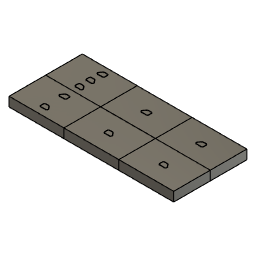
AD_mold_20200226_wide v4 (Autodesk Fusion 360 design; units mm, degrees)
Autodesk Fusion 360 part; units mm, degrees
note: some values were not read from the file. Chosen so that the rebuilt part matches the saved one: which bodies a step acts on.
sketch "Sketch1" plane through (0, 0, 0) normal (0, 1, 0) x (1, 0, 0)
  line L0 (-37.5181, 150.0315) -> (37.4819, 150.0315)
  line L1 (37.4819, 150.0315) -> (37.4819, -149.9685)
  line L2 (37.4819, -149.9685) -> (-37.5181, -149.9685)
  line L3 (-37.5181, -149.9685) -> (-37.5181, 150.0315)
  line L4 (-37.5181, -50.0913) -> (37.4819, -50.0913)
  line L5 (37.4819, -50.0913) -> (37.4819, -100.0913)
  line L6 (37.4819, -100.0913) -> (-37.5181, -100.0913)
  line L7 (-37.5181, -100.0913) -> (-37.5181, -50.0913)
  line L8 (-37.5181, -0.0913) -> (37.4819, -0.0913)
  line L9 (-37.5181, -50.0913) -> (-37.5181, -0.0913)
  line L10 (37.4819, -50.0913) -> (-37.5181, -50.0913)
  line L11 (37.4819, -0.0913) -> (37.4819, -50.0913)
  line L12 (37.4819, -100.0913) -> (-37.5181, -100.0913)
  line L13 (-37.5181, -150.0913) -> (-37.5181, -100.0913)
  line L14 (37.4819, -150.0913) -> (-37.5181, -150.0913)
  line L15 (37.4819, -100.0913) -> (37.4819, -150.0913)
  line L16 (-37.5181, 49.9087) -> (37.4819, 49.9087)
  line L17 (-37.5181, -0.0913) -> (-37.5181, 49.9087)
  line L18 (37.4819, -0.0913) -> (-37.5181, -0.0913)
  line L19 (37.4819, 49.9087) -> (37.4819, -0.0913)
  line L20 (-37.5181, 99.9087) -> (37.4819, 99.9087)
  line L21 (37.4819, 99.9087) -> (37.4819, 49.9087)
  line L22 (-37.5181, 49.9087) -> (37.4819, 49.9087)
  line L23 (-37.5181, 49.9087) -> (-37.5181, 99.9087)
  line L24 (37.4819, 149.9087) -> (37.4819, 99.9087)
  line L25 (-37.5181, 99.9087) -> (-37.5181, 149.9087)
  line L26 (-3.211, -128.2452) -> (3.289, -128.2452)
  arc A0 (3.289, -128.2452) -> (4.789, -126.7452) centre (3.289, -126.7452) ccw
  line L27 (4.789, -126.7452) -> (4.789, -123.3452)
  arc A1 (4.789, -123.3452) -> (3.289, -121.8452) centre (3.289, -123.3452) ccw
  line L28 (3.289, -121.8452) -> (-0.4902, -121.8452)
  arc A2 (-0.4902, -121.8452) -> (-1.6614, -122.408) centre (-0.4902, -123.3452) ccw
  line L29 (-4.3822, -125.808) -> (-1.6614, -122.408)
  arc A3 (-4.3822, -125.808) -> (-4.711, -126.7452) centre (-3.211, -126.7452) ccw
  arc A4 (-4.711, -126.7452) -> (-3.211, -128.2452) centre (-3.211, -126.7452) ccw
  line L30 (-3.211, -28.2452) -> (3.289, -28.2452)
  arc A5 (3.289, -28.2452) -> (4.789, -26.7452) centre (3.289, -26.7452) ccw
  line L31 (4.789, -26.7452) -> (4.789, -23.3452)
  arc A6 (4.789, -23.3452) -> (3.289, -21.8452) centre (3.289, -23.3452) ccw
  line L32 (3.289, -21.8452) -> (-0.4902, -21.8452)
  arc A7 (-0.4902, -21.8452) -> (-1.6614, -22.408) centre (-0.4902, -23.3452) ccw
  line L33 (-4.3822, -25.808) -> (-1.6614, -22.408)
  arc A8 (-4.3822, -25.808) -> (-4.711, -26.7452) centre (-3.211, -26.7452) ccw
  arc A9 (-4.711, -26.7452) -> (-3.211, -28.2452) centre (-3.211, -26.7452) ccw
  line L34 (4.789, 138.2548) -> (4.789, 141.6548)
  arc A10 (3.289, 136.7548) -> (4.789, 138.2548) centre (3.289, 138.2548) ccw
  line L35 (-3.211, 136.7548) -> (3.289, 136.7548)
  arc A11 (-4.711, 138.2548) -> (-3.211, 136.7548) centre (-3.211, 138.2548) ccw
  arc A12 (-4.3822, 139.192) -> (-4.711, 138.2548) centre (-3.211, 138.2548) ccw
  line L36 (-4.3822, 139.192) -> (-1.6614, 142.592)
  arc A13 (-0.4902, 143.1548) -> (-1.6614, 142.592) centre (-0.4902, 141.6548) ccw
  line L37 (3.289, 143.1548) -> (-0.4902, 143.1548)
  arc A14 (4.789, 141.6548) -> (3.289, 143.1548) centre (3.289, 141.6548) ccw
  line L38 (4.789, 86.2548) -> (4.789, 89.6548)
  arc A15 (3.289, 84.7548) -> (4.789, 86.2548) centre (3.289, 86.2548) ccw
  line L39 (-3.211, 84.7548) -> (3.289, 84.7548)
  arc A16 (-4.711, 86.2548) -> (-3.211, 84.7548) centre (-3.211, 86.2548) ccw
  arc A17 (-4.3822, 87.192) -> (-4.711, 86.2548) centre (-3.211, 86.2548) ccw
  line L40 (-4.3822, 87.192) -> (-1.6614, 90.592)
  arc A18 (-0.4902, 91.1548) -> (-1.6614, 90.592) centre (-0.4902, 89.6548) ccw
  line L41 (3.289, 91.1548) -> (-0.4902, 91.1548)
  arc A19 (4.789, 89.6548) -> (3.289, 91.1548) centre (3.289, 89.6548) ccw
  arc A20 (3.1599, 59.3879) -> (4.6599, 60.8879) centre (3.1599, 60.8879) ccw
  arc A21 (4.6599, 60.8879) -> (4.331, 61.8251) centre (3.1599, 60.8879) ccw
  line L42 (4.331, 61.8251) -> (1.6102, 65.2251)
  arc A22 (1.6102, 65.2251) -> (0.4391, 65.7879) centre (0.4391, 64.2879) ccw
  line L43 (-3.3401, 65.7879) -> (0.4391, 65.7879)
  arc A23 (-3.3401, 65.7879) -> (-4.8401, 64.2879) centre (-3.3401, 64.2879) ccw
  line L44 (-4.8401, 60.8879) -> (-4.8401, 64.2879)
  arc A24 (-4.8401, 60.8879) -> (-3.3401, 59.3879) centre (-3.3401, 60.8879) ccw
  line L45 (3.1599, 59.3879) -> (-3.3401, 59.3879)
  arc A25 (3.1599, 106.7879) -> (4.6599, 108.2879) centre (3.1599, 108.2879) ccw
  arc A26 (4.6599, 108.2879) -> (4.331, 109.2251) centre (3.1599, 108.2879) ccw
  line L46 (4.331, 109.2251) -> (1.6102, 112.6251)
  arc A27 (1.6102, 112.6251) -> (0.4391, 113.1879) centre (0.4391, 111.6879) ccw
  line L47 (-3.3401, 113.1879) -> (0.4391, 113.1879)
  arc A28 (-3.3401, 113.1879) -> (-4.8401, 111.6879) centre (-3.3401, 111.6879) ccw
  line L48 (-4.8401, 108.2879) -> (-4.8401, 111.6879)
  arc A29 (-4.8401, 108.2879) -> (-3.3401, 106.7879) centre (-3.3401, 108.2879) ccw
  line L49 (3.1599, 106.7879) -> (-3.3401, 106.7879)
  arc A30 (3.1599, 121.7879) -> (4.6599, 123.2879) centre (3.1599, 123.2879) ccw
  arc A31 (4.6599, 123.2879) -> (4.331, 124.2251) centre (3.1599, 123.2879) ccw
  line L50 (4.331, 124.2251) -> (1.6102, 127.6251)
  arc A32 (1.6102, 127.6251) -> (0.4391, 128.1879) centre (0.4391, 126.6879) ccw
  line L51 (-3.3401, 128.1879) -> (0.4391, 128.1879)
  arc A33 (-3.3401, 128.1879) -> (-4.8401, 126.6879) centre (-3.3401, 126.6879) ccw
  line L52 (-4.8401, 123.2879) -> (-4.8401, 126.6879)
  arc A34 (-4.8401, 123.2879) -> (-3.3401, 121.7879) centre (-3.3401, 123.2879) ccw
  line L53 (3.1599, 121.7879) -> (-3.3401, 121.7879)
  arc A35 (3.1599, 21.7879) -> (4.6599, 23.2879) centre (3.1599, 23.2879) ccw
  arc A36 (4.6599, 23.2879) -> (4.331, 24.2251) centre (3.1599, 23.2879) ccw
  line L54 (4.331, 24.2251) -> (1.6102, 27.6251)
  arc A37 (1.6102, 27.6251) -> (0.4391, 28.1879) centre (0.4391, 26.6879) ccw
  line L55 (-3.3401, 28.1879) -> (0.4391, 28.1879)
  arc A38 (-3.3401, 28.1879) -> (-4.8401, 26.6879) centre (-3.3401, 26.6879) ccw
  line L56 (-4.8401, 23.2879) -> (-4.8401, 26.6879)
  arc A39 (-4.8401, 23.2879) -> (-3.3401, 21.7879) centre (-3.3401, 23.2879) ccw
  line L57 (3.1599, 21.7879) -> (-3.3401, 21.7879)
  arc A40 (3.1599, -78.2121) -> (4.6599, -76.7121) centre (3.1599, -76.7121) ccw
  arc A41 (4.6599, -76.7121) -> (4.331, -75.7749) centre (3.1599, -76.7121) ccw
  line L58 (4.331, -75.7749) -> (1.6102, -72.3749)
  arc A42 (1.6102, -72.3749) -> (0.4391, -71.8121) centre (0.4391, -73.3121) ccw
  line L59 (-3.3401, -71.8121) -> (0.4391, -71.8121)
  arc A43 (-3.3401, -71.8121) -> (-4.8401, -73.3121) centre (-3.3401, -73.3121) ccw
  line L60 (-4.8401, -76.7121) -> (-4.8401, -73.3121)
  arc A44 (-4.8401, -76.7121) -> (-3.3401, -78.2121) centre (-3.3401, -76.7121) ccw
  line L61 (3.1599, -78.2121) -> (-3.3401, -78.2121)
  line L62 (-4.6921, 139.44) -> (-1.9713, 142.84)
  arc A45 (-0.4902, 143.5517) -> (-1.9713, 142.84) centre (-0.4902, 141.6548) ccw
  line L63 (3.289, 143.5517) -> (-0.4902, 143.5517)
  arc A46 (5.1859, 141.6548) -> (3.289, 143.5517) centre (3.289, 141.6548) ccw
  line L64 (5.1859, 138.2548) -> (5.1859, 141.6548)
  arc A47 (3.289, 136.3579) -> (5.1859, 138.2548) centre (3.289, 138.2548) ccw
  line L65 (-3.211, 136.3579) -> (3.289, 136.3579)
  arc A48 (-5.1079, 138.2548) -> (-3.211, 136.3579) centre (-3.211, 138.2548) ccw
  arc A49 (-4.6921, 139.44) -> (-5.1079, 138.2548) centre (-3.211, 138.2548) ccw
  line L66 (-3.3401, 128.5848) -> (0.4391, 128.5848)
  arc A50 (1.9201, 127.8731) -> (0.4391, 128.5848) centre (0.4391, 126.6879) ccw
  line L67 (4.6409, 124.4731) -> (1.9201, 127.8731)
  arc A51 (5.0568, 123.2879) -> (4.6409, 124.4731) centre (3.1599, 123.2879) ccw
  arc A52 (3.1599, 121.391) -> (5.0568, 123.2879) centre (3.1599, 123.2879) ccw
  line L68 (3.1599, 121.391) -> (-3.3401, 121.391)
  arc A53 (-5.237, 123.2879) -> (-3.3401, 121.391) centre (-3.3401, 123.2879) ccw
  line L69 (-5.237, 123.2879) -> (-5.237, 126.6879)
  arc A54 (-3.3401, 128.5848) -> (-5.237, 126.6879) centre (-3.3401, 126.6879) ccw
  line L70 (-3.3401, 113.5848) -> (0.4391, 113.5848)
  arc A55 (1.9201, 112.8731) -> (0.4391, 113.5848) centre (0.4391, 111.6879) ccw
  line L71 (4.6409, 109.4731) -> (1.9201, 112.8731)
  arc A56 (5.0568, 108.2879) -> (4.6409, 109.4731) centre (3.1599, 108.2879) ccw
  arc A57 (3.1599, 106.391) -> (5.0568, 108.2879) centre (3.1599, 108.2879) ccw
  line L72 (3.1599, 106.391) -> (-3.3401, 106.391)
  arc A58 (-5.237, 108.2879) -> (-3.3401, 106.391) centre (-3.3401, 108.2879) ccw
  line L73 (-5.237, 108.2879) -> (-5.237, 111.6879)
  arc A59 (-3.3401, 113.5848) -> (-5.237, 111.6879) centre (-3.3401, 111.6879) ccw
  line L74 (-4.6921, 87.44) -> (-1.9713, 90.84)
  arc A60 (-0.4902, 91.5517) -> (-1.9713, 90.84) centre (-0.4902, 89.6548) ccw
  line L75 (3.289, 91.5517) -> (-0.4902, 91.5517)
  arc A61 (5.1859, 89.6548) -> (3.289, 91.5517) centre (3.289, 89.6548) ccw
  line L76 (5.1859, 86.2548) -> (5.1859, 89.6548)
  arc A62 (3.289, 84.3579) -> (5.1859, 86.2548) centre (3.289, 86.2548) ccw
  line L77 (-3.211, 84.3579) -> (3.289, 84.3579)
  arc A63 (-5.1079, 86.2548) -> (-3.211, 84.3579) centre (-3.211, 86.2548) ccw
  arc A64 (-4.6921, 87.44) -> (-5.1079, 86.2548) centre (-3.211, 86.2548) ccw
  line L78 (-3.3401, 66.1848) -> (0.4391, 66.1848)
  arc A65 (1.9201, 65.4731) -> (0.4391, 66.1848) centre (0.4391, 64.2879) ccw
  line L79 (4.6409, 62.0731) -> (1.9201, 65.4731)
  arc A66 (5.0568, 60.8879) -> (4.6409, 62.0731) centre (3.1599, 60.8879) ccw
  arc A67 (3.1599, 58.991) -> (5.0568, 60.8879) centre (3.1599, 60.8879) ccw
  line L80 (3.1599, 58.991) -> (-3.3401, 58.991)
  arc A68 (-5.237, 60.8879) -> (-3.3401, 58.991) centre (-3.3401, 60.8879) ccw
  line L81 (-5.237, 60.8879) -> (-5.237, 64.2879)
  arc A69 (-3.3401, 66.1848) -> (-5.237, 64.2879) centre (-3.3401, 64.2879) ccw
  line L82 (-3.3401, 28.5848) -> (0.4391, 28.5848)
  arc A70 (1.9201, 27.8731) -> (0.4391, 28.5848) centre (0.4391, 26.6879) ccw
  line L83 (4.6409, 24.4731) -> (1.9201, 27.8731)
  arc A71 (5.0568, 23.2879) -> (4.6409, 24.4731) centre (3.1599, 23.2879) ccw
  arc A72 (3.1599, 21.391) -> (5.0568, 23.2879) centre (3.1599, 23.2879) ccw
  line L84 (3.1599, 21.391) -> (-3.3401, 21.391)
  arc A73 (-5.237, 23.2879) -> (-3.3401, 21.391) centre (-3.3401, 23.2879) ccw
  line L85 (-5.237, 23.2879) -> (-5.237, 26.6879)
  arc A74 (-3.3401, 28.5848) -> (-5.237, 26.6879) centre (-3.3401, 26.6879) ccw
  arc A75 (5.1859, -23.3452) -> (3.289, -21.4483) centre (3.289, -23.3452) ccw
  line L86 (3.289, -21.4483) -> (-0.4902, -21.4483)
  arc A76 (-0.4902, -21.4483) -> (-1.9713, -22.16) centre (-0.4902, -23.3452) ccw
  line L87 (-4.6921, -25.56) -> (-1.9713, -22.16)
  arc A77 (-4.6921, -25.56) -> (-5.1079, -26.7452) centre (-3.211, -26.7452) ccw
  arc A78 (-5.1079, -26.7452) -> (-3.211, -28.6421) centre (-3.211, -26.7452) ccw
  line L88 (-3.211, -28.6421) -> (3.289, -28.6421)
  arc A79 (3.289, -28.6421) -> (5.1859, -26.7452) centre (3.289, -26.7452) ccw
  line L89 (5.1859, -26.7452) -> (5.1859, -23.3452)
  line L90 (-3.3401, -71.4152) -> (0.4391, -71.4152)
  arc A80 (1.9201, -72.1269) -> (0.4391, -71.4152) centre (0.4391, -73.3121) ccw
  line L91 (4.6409, -75.5269) -> (1.9201, -72.1269)
  arc A81 (5.0568, -76.7121) -> (4.6409, -75.5269) centre (3.1599, -76.7121) ccw
  arc A82 (3.1599, -78.609) -> (5.0568, -76.7121) centre (3.1599, -76.7121) ccw
  line L92 (3.1599, -78.609) -> (-3.3401, -78.609)
  arc A83 (-5.237, -76.7121) -> (-3.3401, -78.609) centre (-3.3401, -76.7121) ccw
  line L93 (-5.237, -76.7121) -> (-5.237, -73.3121)
  arc A84 (-3.3401, -71.4152) -> (-5.237, -73.3121) centre (-3.3401, -73.3121) ccw
  line L94 (-4.6921, -125.56) -> (-1.9713, -122.16)
  arc A85 (-0.4902, -121.4483) -> (-1.9713, -122.16) centre (-0.4902, -123.3452) ccw
  line L95 (3.289, -121.4483) -> (-0.4902, -121.4483)
  arc A86 (5.1859, -123.3452) -> (3.289, -121.4483) centre (3.289, -123.3452) ccw
  line L96 (5.1859, -126.7452) -> (5.1859, -123.3452)
  arc A87 (3.289, -128.6421) -> (5.1859, -126.7452) centre (3.289, -126.7452) ccw
  line L97 (-3.211, -128.6421) -> (3.289, -128.6421)
  arc A88 (-5.1079, -126.7452) -> (-3.211, -128.6421) centre (-3.211, -126.7452) ccw
  arc A89 (-4.6921, -125.56) -> (-5.1079, -126.7452) centre (-3.211, -126.7452) ccw
  dimension "d1" = 75
  dimension "d2" = 300
  dimension "d3" = 50
  dimension "d4" = 50
  dimension "d5" = 50
  dimension "d6" = 50
  dimension "d7" = 50
  dimension "d8" = 50
  dimension "d9" = 0.3969
  dimension "d10" = 0.3969
  dimension "d11" = 0.3969
  dimension "d12" = 0.3969
  dimension "d13" = 0.3969
  dimension "d14" = 0.3969
  dimension "d15" = 0.3969
  dimension "d16" = 0.3969
  dimension "d17" = 0.3969
  constraint horizontal L0
  constraint vertical L1
  constraint horizontal L2
  constraint vertical L3
  constraint horizontal L4
  constraint vertical L5
  constraint horizontal L6
  constraint vertical L7
  constraint coincident L3 L4.start
  constraint vertical L11
  constraint horizontal L10
  constraint vertical L9
  constraint vertical L15
  constraint horizontal L14
  constraint vertical L13
  constraint horizontal L12
  constraint horizontal L16
  constraint vertical L19
  constraint vertical L17
  constraint horizontal L22
  constraint horizontal L20
  constraint vertical L21
  constraint vertical L23
  constraint vertical L24
  constraint vertical L25
  constraint horizontal L43
  constraint tangent L43 A23
  constraint tangent A22 L43
  constraint horizontal L45
  constraint concentric A20 A21
  constraint tangent A21 L42
  constraint horizontal L47
  constraint tangent L47 A28
  constraint tangent A27 L47
  constraint horizontal L49
  constraint concentric A25 A26
  constraint tangent A26 L46
  constraint horizontal L51
  constraint tangent L51 A33
  constraint tangent A32 L51
  constraint horizontal L53
  constraint concentric A30 A31
  constraint tangent A31 L50
  constraint horizontal L55
  constraint tangent L55 A38
  constraint tangent A37 L55
  constraint horizontal L57
  constraint concentric A35 A36
  constraint tangent A36 L54
  constraint horizontal L59
  constraint tangent L59 A43
  constraint tangent A42 L59
  constraint horizontal L61
  constraint concentric A40 A41
  constraint tangent A41 L58
  measures "d1" distance of L0.start L0.end
  measures "d2" distance of L0.end L1.end
  measures "d3" distance of L4.start L6.end
  measures "d4" distance of L4.start L8.start
  measures "d5" distance of L13.start L6.end
  measures "d6" distance of L16.start L8.start
  measures "d7" distance of L16.start L20.start
  measures "d8" distance of L20.start L25.end
extrude "Extrude1" add sketch "Sketch1" along normal blind 12.7 contours L0 L1 L3 L20 L24 L25 | L1 L3 L16 L20 L21 L22 L23 | L1 L3 L8 L16 L17 L18 L19 L22 | L1 L3 L4 L8 L9 L10 L11 L18 | L1 L3 L4 L5 L6 L7 L10 L12 | L1 L2 L3 L6 L12 L13 L15 | L26 A0 L27 A1 L28 A2 L29 A3 A4 | L30 A5 L31 A6 L32 A7 L33 A8 A9 | L34 A10 L35 A11 A12 L36 A13 L37 A14 | L38 A15 L39 A16 A17 L40 A18 L41 A19 | A20 A21 L42 A22 L43 A23 L44 A24 L45 | A25 A26 L46 A27 L47 A28 L48 A29 L49 | A30 A31 L50 A32 L51 A33 L52 A34 L53 | A35 A36 L54 A37 L55 A38 L56 A39 L57 | A40 A41 L58 A42 L59 A43 L60 A44 L61 makes body 1 at (0.9932, 4.2333, -106.7879) makes body 2 at (-1.0444, 4.2333, 128.2452) makes body 3 at (26.7166, 0, 7.7608) makes body 4 at (0.9932, 4.2333, -21.7879) makes body 5 at (0.9932, 4.2333, -121.7879) makes body 6 at (-1.0444, 4.2333, -84.7548) makes body 7 at (0.9932, 4.2333, 78.2121) makes body 8 at (-1.0444, 4.2333, 28.2452) makes body 9 at (0.9932, 4.2333, -59.3879) makes body 10 at (-1.0444, 4.2333, -136.7548)
extrude "Extrude2" add sketch "Sketch1" along normal blind 10.7156 contours L62 A45 L63 A46 L64 A47 L65 A48 A49 | L66 A50 L67 A51 A52 L68 A53 L69 A54 | L70 A55 L71 A56 A57 L72 A58 L73 A59 bodies 1 3 5 10
extrude "Extrude3" add sketch "Sketch1" along normal blind 10.7156 contours L74 A60 L75 A61 L76 A62 L77 A63 A64 | L78 A65 L79 A66 A67 L80 A68 L81 A69 | L82 A70 L83 A71 A72 L84 A73 L85 A74 | A75 L86 A76 L87 A77 A78 L88 A79 L89 | L90 A80 L91 A81 A82 L92 A83 L93 A84 bodies 1 4 6 7 8 9
extrude "Extrude4" add sketch "Sketch1" along normal blind 10.7156 contours L94 A85 L95 A86 L96 A87 L97 A88 A89 bodies 1 2
extrude "Extrude5" add sketch "Sketch1" along normal blind 0.5 separate body contours L62 A45 L63 A46 L64 A47 L65 A48 A49 | L66 A50 L67 A51 A52 L68 A53 L69 A54 | L70 A55 L71 A56 A57 L72 A58 L73 A59 makes body 11 at (1.1223, 0, -136.4902) makes body 12 at (0.9932, 0, -121.5233) makes body 13 at (0.9932, 0, -106.5233)
extrude "Extrude6" add sketch "Sketch1" along normal blind 0.5 separate body contours L62 A45 L63 A46 L64 A47 L65 A48 A49 makes body 14
extrude "Extrude7" add 5 faces at (1.1223, 10.7156, -136.4902) (0.9932, 10.7156, -121.5233) (0.9932, 10.7156, -106.5233) (-1.0444, 10.7156, -84.6225) (0.9932, 10.7156, -59.1233) along direction (0, 1, 0) blind 0.484 on bodies 1 bodies 1
extrude "Extrude8" add 4 faces at (-1.1735, 10.7156, -21.6556) (-1.0444, 10.7156, 28.5098) (-1.1735, 10.7156, 78.4767) (1.1223, 10.7156, 128.5098) along direction (0, 1, 0) blind 0.484 on bodies 1 bodies 1
split "Split1" by curves path "Sketch1" along L7 L4 L5 L6 bodies 1 makes body 15 at (-12.5181, 0, 116.717) makes body 16 at (-12.5181, 0, -83.3239)
split "Split2" by curves path "Sketch1" along L17 L16 L19 L18 bodies 16 makes body 17 at (12.4819, 0, -116.6572) makes body 18 at (-12.5181, 0, 33.4246)
split "Split3" by curves path "Sketch1" along L23 L20 L21 bodies 17 makes body 19 at (-12.5181, 0, -133.3239)
move_body "Move1" bodies 15 to x (1, 0, 0) y (0, 1, 0) z (0, 0, 1) at (75, 0, -250)
move_face "MoveFace1" by (75, 0, 0) 1 faces at (26.6717, 12.7, 75.5835) on bodies 1
move_body "Move2" bodies 1 to x (1, 0, 0) y (0, 1, 0) z (0, 0, 1) at (75, 0, 0)
move_body "Move3" bodies 1 to x (1, 0, 0) y (0, 1, 0) z (0, 0, 1) at (0, 0, -150)
move_body "Move4" bodies 18 to x (1, 0, 0) y (0, 1, 0) z (0, 0, 1) at (150, 0, 0)
move_body "Move5" bodies 18 to x (1, 0, 0) y (0, 1, 0) z (0, 0, 1) at (0, 0, -150)
move_body "Move6" bodies 16 to x (1, 0, 0) y (0, 1, 0) z (0, 0, 1) at (150, 0, -50)
move_body "Move7" bodies 16 15 18 17 11 14 12 19 13 1 to x (1, 0, 0) y (0, 1, 0) z (0, 0, 1) at (0, 0, 100)
move_body "Move8" bodies 12 17 19 13 14 1 11 18 16 15 to x (1, 0, 0) y (0, 1, 0) z (0, 0, 1) at (-75, 0, 0)
sketch "Sketch5" plane through (0.039, 0, -139.9548) normal (0, 1, 0) x (1, 0, 0)
sketch "Sketch2" plane through (-0.0901, 0, 75.0121) normal (0, 1, 0) x (1, 0, 0)
sketch "Sketch3" plane through (0, 0, 0) normal (0, 1, 0) x (1, 0, 0)
sketch "Sketch4" plane through (0, 0, 0) normal (0, 1, 0) x (1, 0, 0)
